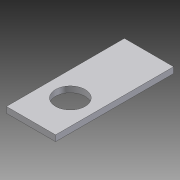
# Autodesk Inventor part: BOTTOM
Saved by Autodesk Inventor 2012 SP2 (Build 160219200, 219)
## iProperties
Created: 2013-03-12
Part Number: BOTTOM
Material: Default
Document SubType Name: Modeling
Designer: blacki
Density: 1 g/cm^3
Author: blacki
Autodesk Inventor part; units mm, degrees
ref_plane "YZ Plane" through (0, 0, 0) normal (1, 0, 0) x (0, 1, 0)
ref_plane "XZ Plane" through (0, 0, 0) normal (0, 1, 0) x (-1, 0, 0)
ref_plane "XY Plane" through (0, 0, 0) normal (0, 0, 1) x (1, 0, 0)
sketch "Sketch1" plane through (0, 0, 0) normal (0, 0, 1) x (1, 0, 0)
  line L0 (-25, 70) -> (25, 70)
  line L1 (25, 70) -> (25, -70)
  line L2 (25, -70) -> (-25, -70)
  line L3 (-25, -70) -> (-25, 70)
  line L4 (-25, 0) -> (25, 0) construction
  point P0 (0, 0)
  point P1 (0, 0)
  dimension "d0" = 50
  dimension "d1" = 140
  constraints: 10 end point, 3 midpoint, 2 parallel, 1 coincident, 1 horizontal, 1 perpendicular
  measures "d0" distance of L1.end L2.end
  measures "d1" distance of L0.end L1.end
extrude "Extrusion1" add sketch "Sketch1" along normal blind 6
sketch "Sketch2" plane through (0, 0, 0) normal (0, 0, -1) x (-1, 0, 0)
  line L0 (25, 70) -> (-25, 70) projected
  line L1 (-25, -70) -> (25, -70) projected
  line L2 (25, -70) -> (25, 70) projected
  line L3 (0, 70) -> (0, -15) construction
  point P0 (0, 0)
  dimension "d4" = 55
  constraints: 2 end point, 1 coincident, 1 midpoint, 1 parallel
  measures "d4" distance from line of L1 point (0, -15)
hole "Hole1" at (0, -15, 0) direction (0, 0, 1) diameter 30 end through all
sketch "Sketch3" plane through (0, 0, 6) normal (0, 0, 1) x (1, 0, 0)
  circle A0 centre (0, -15) radius 15 projected
  line L0 (25, 70) -> (25, -70) projected
  line L1 (-25, 70) -> (25, 70) projected
  line L2 (-25, -70) -> (-25, 70) projected
  line L3 (25, -70) -> (-25, -70) projected
  circle A1 centre (-13.8351, 16.5) radius 1.5 projected
  circle A2 centre (21.1649, 40) radius 1.5 projected
  point P0 (0, 0)
  constraints: 2 coincident
hole "Hole2" at (-13.8351, 16.5, 6) at (21.1649, 40, 6) direction (0, 0, -1) diameter 3 end through all
sketch "Sketch4" plane through (0, 0, 0) normal (0, 0, -1) x (-1, 0, 0)
  line L0 (25, 70) -> (-25, 70) projected
  line L1 (-25, 70) -> (-25, -70) projected
  line L2 (-25, 64) -> (-10, 64) projected
  line L3 (-10, 70) -> (-10, 64) projected
  line L4 (-25, 70) -> (-10, 70) projected
  line L5 (-25, 70) -> (-25, 64) projected
  line L6 (10, 64) -> (25, 64) projected
  line L7 (25, 70) -> (25, 64) projected
  line L8 (10, 70) -> (25, 70) projected
  line L9 (10, 70) -> (10, 64) projected
  point P0 (0, 0)
extrude "Extrusion2" cut sketch "Sketch4" against normal up to next
sketch "Sketch5" plane through (0, 0, 0) normal (0, 0, -1) x (-1, 0, 0)
  circle A0 centre (0, -15) radius 15 projected
  line L0 (-16, -35) -> (16, -35) construction
  line L1 (16, -35) -> (16, -59) construction
  line L2 (16, -59) -> (-16, -59) construction
  line L3 (-16, -59) -> (-16, -35) construction
  line L4 (-16, -47) -> (16, -47) construction
  circle A1 centre (0, -47) radius 11.5 construction
  line L5 (-16, -35) -> (-11.5, -35) construction
  line L6 (-11.5, -35) -> (-11.5, -43) construction
  line L7 (-11.5, -43) -> (-16, -43) construction
  line L8 (-16, -43) -> (-16, -35) construction
  line L9 (11.5, -35) -> (16, -35) construction
  line L10 (16, -35) -> (16, -43) construction
  line L11 (16, -43) -> (11.5, -43) construction
  line L12 (11.5, -43) -> (11.5, -35) construction
  line L13 (-16, -51) -> (-11.5, -51) construction
  line L14 (-11.5, -51) -> (-11.5, -59) construction
  line L15 (-11.5, -59) -> (-16, -59) construction
  line L16 (-16, -59) -> (-16, -51) construction
  line L17 (11.5, -51) -> (16, -51) construction
  line L18 (16, -51) -> (16, -59) construction
  line L19 (16, -59) -> (11.5, -59) construction
  line L20 (11.5, -59) -> (11.5, -51) construction
  line L21 (-16, -35) -> (16, -35)
  line L22 (16, -35) -> (16, -43)
  line L23 (16, -43) -> (11.5, -43)
  line L24 (11.5, -43) -> (11.5, -51)
  line L25 (11.5, -51) -> (16, -51)
  line L26 (16, -51) -> (16, -59)
  line L27 (16, -59) -> (-16, -59)
  line L28 (-16, -59) -> (-16, -51)
  line L29 (-16, -51) -> (-11.5, -51)
  line L30 (-11.5, -51) -> (-11.5, -43)
  line L31 (-16, -43) -> (-11.5, -43)
  line L32 (-16, -43) -> (-16, -35)
  point P0 (0, 0)
  dimension "d21" = 24
  dimension "d22" = 32
  dimension "d23" = 20
  dimension "d24" = 16
  dimension "d25" = 23
  dimension "d26" = 4
  dimension "d27" = 4.5
  dimension "d28" = 8
  dimension "d31" = 27.5
  dimension "d34" = 16
  constraints: 66 end point, 13 perpendicular, 4 parallel, 3 horizontal, 3 midpoint, 1 centre point, 1 collinear, 1 tangent, 1 vertical, 1 vertical alignment, 24 other
  measures "d21" distance of L0.end L1.end
  measures "d22" distance of L1.end L2.end
  measures "d23" distance from line of point (0, -15) L0
  measures "d24" distance from line of point (0, -15) L3
  measures "d25" diameter of A1
  measures "d26" distance between parallel lines of L4 L7
  measures "d27" distance of L6.end L7.end
  measures "d28" distance of L5.end L6.end
  measures "d31" distance of L6.end L11.start
  measures "d34" distance of L6.end L15.start
extrude "Extrusion3" cut sketch "Sketch5" against normal up to next contours L21 L22 L23 L24 L25 L26 L27 L28 L29 L30 L31 L32
sketch "Sketch6" plane through (0, 0, 0) normal (0, 0, -1) x (-1, 0, 0)
  line L0 (-16, -35) -> (16, -35) projected
  line L1 (16, -59) -> (-16, -59) projected
  line L2 (-10, 70) -> (-10, 64) projected
  line L3 (-14, -47) -> (14, -47) construction
  line L4 (0, -35) -> (0, -59) construction
  point P0 (0, 0)
  point P1 (0, -47)
  dimension "d39" = 28
  dimension "d40" = 14
  constraints: 4 end point, 4 midpoint, 2 coincident, 1 perpendicular
  measures "d39" distance of L3.start L3.end
  measures "d40" distance from line of L4 L3.start
hole "Hole3" at (-14, -47, 0) at (14, -47, 0) direction (0, 0, 1) diameter 2.5 end through all
fillet "Fillet1" radius 2 8 edges at (11.5, -51, 3) (11.5, -43, 3) (16, -43, 3) (16, -51, 3) (-11.5, -51, 3) (-11.5, -43, 3) (-16, -43, 3) (-16, -51, 3) curvature continuous yes
equation "\"d24\" = 0.5 * d22"
equation "\"d31\" = d22 - d27"
equation "\"d34\" = d21 - d28"
equation "\"d40\" = 0.5 * d39"
body "Solid1"
